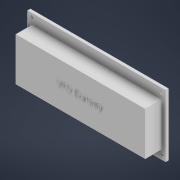
# Autodesk Inventor part: VFD_Dummy
Saved by Autodesk Inventor 2021.1 (Build 251245010, 245A)
## iProperties
Created: 2020-11-27
Part Number: VFD_Dummy
Material: Generic
Document SubType Name: Modeling
Designer: Alex
Density: 1 g/cm^3
Appearance: Default
Author: Alex
Autodesk Inventor part; units mm, degrees
ref_plane "YZ Plane" through (0, 0, 0) normal (1, 0, 0) x (0, 1, 0)
ref_plane "XZ Plane" through (0, 0, 0) normal (0, 1, 0) x (-1, 0, 0)
ref_plane "XY Plane" through (0, 0, 0) normal (0, 0, 1) x (1, 0, 0)
sketch "Sketch1" plane through (0, 0, 0) normal (0, 0, 1) x (1, 0, 0)
  line L0 (-40, 18) -> (40, 18)
  line L1 (40, 18) -> (40, -18)
  line L2 (40, -18) -> (-40, -18)
  line L3 (-40, -18) -> (-40, 18)
  point P0 (0, 0)
  point P1 (0, 18)
  point P2 (-40, 0)
  dimension "d0" = 36
  dimension "d1" = 80
  constraints: 8 end point, 2 midpoint, 2 parallel, 1 horizontal, 1 horizontal alignment, 1 perpendicular, 1 vertical alignment
  measures "d0" distance of L2.end L0.start
  measures "d1" distance of L0.start L0.end
extrude "Extrusion1" add sketch "Sketch1" along normal blind 1.6
sketch "Sketch2" plane through (0, 0, 1.6) normal (0, 0, 1) x (1, 0, 0)
  line L0 (-40, -18) -> (40, -18) construction
  line L1 (40, -18) -> (40, 18) construction
  line L2 (40, 18) -> (-40, 18) construction
  line L3 (-40, 18) -> (-40, -18) construction
  point P0 (0, 0)
  point P1 (-37.5, 15.5)
  point P2 (-37.5, -15.5)
  point P3 (37.5, -15.5)
  point P4 (37.5, 15.5)
  dimension "d4" = 2.5
  dimension "d5" = 2.5
  dimension "d6" = 2.5
  dimension "d7" = 2.5
  constraints: 2 horizontal alignment, 2 vertical alignment
  measures "d4" distance from line of L2 point (-37.5, 15.5)
  measures "d5" distance from line of L3 point (-37.5, 15.5)
  measures "d6" distance from line of L0 point (37.5, -15.5)
  measures "d7" distance from line of L1 point (37.5, -15.5)
hole "Hole1" at (-37.5, 15.5, 1.6) at (-37.5, -15.5, 1.6) at (37.5, -15.5, 1.6) at (37.5, 15.5, 1.6) direction (0, 0, -1) diameter 2.5 depth 5
sketch "Sketch3" plane through (0, 0, 1.6) normal (0, 0, 1) x (1, 0, 0)
  line L0 (-37.5, 11.95) -> (37.5, 11.95)
  line L1 (37.5, 11.95) -> (37.5, -13.05)
  line L2 (37.5, -13.05) -> (-37.5, -13.05)
  line L3 (-37.5, -13.05) -> (-37.5, 11.95)
  line L4 (-40, -18) -> (40, -18) projected
  point P0 (0, 0)
  point P1 (0, 11.95)
  dimension "d15" = 25
  dimension "d16" = 75
  dimension "d17" = 4.95
  constraints: 8 end point, 2 parallel, 1 horizontal, 1 midpoint, 1 perpendicular, 1 vertical alignment
  measures "d15" distance of L2.end L0.start
  measures "d16" distance of L0.start L0.end
  measures "d17" distance between parallel lines of L2 L4
extrude "Extrusion2" add sketch "Sketch3" along normal blind 9.35
sketch "Sketch4" plane through (0, 0, 10.95) normal (0, 0, 1) x (1, 0, 0)
  line L0 (-22.5, 4.45) -> (22.5, 4.45) construction
  line L1 (22.5, 4.45) -> (22.5, -5.55) construction
  line L2 (22.5, -5.55) -> (-22.5, -5.55) construction
  line L3 (-22.5, -5.55) -> (-22.5, 4.45) construction
  line L4 (-37.5, -13.05) -> (37.5, -13.05) construction
  line L5 (37.5, -13.05) -> (37.5, 11.95) construction
  line L6 (37.5, 11.95) -> (-37.5, 11.95) construction
  line L7 (-37.5, 11.95) -> (-37.5, -13.05) construction
  line L8 (37.5, 11.95) -> (-37.5, 11.95) construction
  line L9 (-10.3965, 1.6836) -> (-11.6019, -1.8164)
  line L10 (-11.6019, -1.8164) -> (-12.1039, -1.8164)
  line L11 (-12.1039, -1.8164) -> (-13.3094, 1.6836)
  line L12 (-13.3094, 1.6836) -> (-12.8102, 1.6836)
  line L13 (-12.8102, 1.6836) -> (-11.8402, -1.2236)
  line L14 (-11.8402, -1.2236) -> (-10.8701, 1.6836)
  line L15 (-10.8701, 1.6836) -> (-10.3965, 1.6836)
  line L16 (-7.9686, 1.2695) -> (-9.5966, 1.2695)
  line L17 (-9.5966, 1.2695) -> (-9.5966, 0.2825)
  line L18 (-9.5966, 0.2825) -> (-8.0367, 0.2825)
  line L19 (-8.0367, 0.2825) -> (-8.0367, -0.1316)
  line L20 (-8.0367, -0.1316) -> (-9.5966, -0.1316)
  line L21 (-9.5966, -0.1316) -> (-9.5966, -1.8164)
  line L22 (-9.5966, -1.8164) -> (-10.0618, -1.8164)
  line L23 (-10.0618, -1.8164) -> (-10.0618, 1.6836)
  line L24 (-10.0618, 1.6836) -> (-7.9686, 1.6836)
  line L25 (-7.9686, 1.6836) -> (-7.9686, 1.2695)
  spline S0 degree 2 poles (-4.7919, -0.0692) (-4.7919, -0.5486) (-5.1805, -1.3201) (-5.5067, -1.5356) knots 0 0 0 1 2 2 2
  spline S1 degree 2 poles (-5.5067, -1.5356) (-5.7733, -1.703) (-6.3207, -1.8164) (-6.7462, -1.8164) knots 0 0 0 1 2 2 2
  line L26 (-6.7462, -1.8164) -> (-7.5517, -1.8164)
  line L27 (-7.5517, -1.8164) -> (-7.5517, 1.6836)
  line L28 (-7.5517, 1.6836) -> (-6.7547, 1.6836)
  spline S2 degree 2 poles (-6.7547, 1.6836) (-6.2611, 1.6836) (-5.6996, 1.5361) (-5.501, 1.4056) knots 0 0 0 1 2 2 2
  spline S3 degree 2 poles (-5.501, 1.4056) (-5.1635, 1.1816) (-4.7919, 0.4413) (-4.7919, -0.0692) knots 0 0 0 1 2 2 2
  spline S4 degree 2 poles (-5.2769, -0.0636) (-5.2769, 0.3392) (-5.5436, 0.9093) (-5.8073, 1.0709) knots 0 0 0 1 2 2 2
  spline S5 degree 2 poles (-5.8073, 1.0709) (-5.9945, 1.1816) (-6.4171, 1.2808) (-6.732, 1.2808) knots 0 0 0 1 2 2 2
  line L29 (-6.732, 1.2808) -> (-7.0865, 1.2808)
  line L30 (-7.0865, 1.2808) -> (-7.0865, -1.4137)
  line L31 (-7.0865, -1.4137) -> (-6.732, -1.4137)
  spline S6 degree 2 poles (-6.732, -1.4137) (-6.4228, -1.4137) (-5.9548, -1.3144) (-5.7648, -1.1811) knots 0 0 0 1 2 2 2
  spline S7 degree 2 poles (-5.7648, -1.1811) (-5.5209, -1.0166) (-5.2769, -0.472) (-5.2769, -0.0636) knots 0 0 0 1 2 2 2
  spline S8 degree 2 poles (-0.0241, -0.0692) (-0.0241, -0.5486) (-0.4127, -1.3201) (-0.7389, -1.5356) knots 0 0 0 1 2 2 2
  spline S9 degree 2 poles (-0.7389, -1.5356) (-1.0055, -1.703) (-1.5529, -1.8164) (-1.9783, -1.8164) knots 0 0 0 1 2 2 2
  line L32 (-1.9783, -1.8164) -> (-2.7838, -1.8164)
  line L33 (-2.7838, -1.8164) -> (-2.7838, 1.6836)
  line L34 (-2.7838, 1.6836) -> (-1.9868, 1.6836)
  spline S10 degree 2 poles (-1.9868, 1.6836) (-1.4933, 1.6836) (-0.9317, 1.5361) (-0.7332, 1.4056) knots 0 0 0 1 2 2 2
  spline S11 degree 2 poles (-0.7332, 1.4056) (-0.3957, 1.1816) (-0.0241, 0.4413) (-0.0241, -0.0692) knots 0 0 0 1 2 2 2
  spline S12 degree 2 poles (-0.5091, -0.0636) (-0.5091, 0.3392) (-0.7757, 0.9093) (-1.0395, 1.0709) knots 0 0 0 1 2 2 2
  spline S13 degree 2 poles (-1.0395, 1.0709) (-1.2267, 1.1816) (-1.6493, 1.2808) (-1.9641, 1.2808) knots 0 0 0 1 2 2 2
  line L35 (-1.9641, 1.2808) -> (-2.3187, 1.2808)
  line L36 (-2.3187, 1.2808) -> (-2.3187, -1.4137)
  line L37 (-2.3187, -1.4137) -> (-1.9641, -1.4137)
  spline S14 degree 2 poles (-1.9641, -1.4137) (-1.655, -1.4137) (-1.187, -1.3144) (-0.997, -1.1811) knots 0 0 0 1 2 2 2
  spline S15 degree 2 poles (-0.997, -1.1811) (-0.753, -1.0166) (-0.5091, -0.472) (-0.5091, -0.0636) knots 0 0 0 1 2 2 2
  line L38 (2.4889, -1.8164) -> (2.0464, -1.8164)
  line L39 (2.0464, -1.8164) -> (2.0464, -1.5271)
  spline S16 degree 2 poles (2.0464, -1.5271) (1.8422, -1.7058) (1.4763, -1.8902) (1.2494, -1.8902) knots 0 0 0 1 2 2 2
  spline S17 degree 2 poles (1.2494, -1.8902) (1.0792, -1.8902) (0.7757, -1.7767) (0.6651, -1.6547) knots 0 0 0 1 2 2 2
  spline S18 degree 2 poles (0.6651, -1.6547) (0.5517, -1.5328) (0.4269, -1.1612) (0.4269, -0.8946) knots 0 0 0 1 2 2 2
  line L40 (0.4269, -0.8946) -> (0.4269, 0.81)
  line L41 (0.4269, 0.81) -> (0.8693, 0.81)
  line L42 (0.8693, 0.81) -> (0.8693, -0.6876)
  spline S19 degree 2 poles (0.8693, -0.6876) (0.8693, -0.8974) (0.9005, -1.1726) (0.9544, -1.2747) knots 0 0 0 1 2 2 2
  spline S20 degree 2 poles (0.9544, -1.2747) (1.0083, -1.3768) (1.1927, -1.4704) (1.3657, -1.4704) knots 0 0 0 1 2 2 2
  spline S21 degree 2 poles (1.3657, -1.4704) (1.5273, -1.4704) (1.8932, -1.286) (2.0464, -1.1527) knots 0 0 0 1 2 2 2
  line L43 (2.0464, -1.1527) -> (2.0464, 0.81)
  line L44 (2.0464, 0.81) -> (2.4889, 0.81)
  line L45 (2.4889, 0.81) -> (2.4889, -1.8164)
  line L46 (6.108, -1.8164) -> (6.108, -0.2962)
  spline S22 degree 2 poles (6.108, -0.2962) (6.108, -0.1146) (6.0796, 0.1945) (6.0342, 0.2796) knots 0 0 0 1 2 2 2
  spline S23 degree 2 poles (6.0342, 0.2796) (5.9889, 0.3732) (5.8158, 0.464) (5.6655, 0.464) knots 0 0 0 1 2 2 2
  spline S24 degree 2 poles (5.6655, 0.464) (5.5294, 0.464) (5.2174, 0.2966) (5.0529, 0.1378) knots 0 0 0 1 2 2 2
  spline S25 degree 2 poles (5.0529, 0.1378) (5.0557, 0.0981) (5.0614, -0.0125) (5.0614, -0.0863) knots 0 0 0 1 2 2 2
  line L47 (5.0614, -0.0863) -> (5.0614, -1.8164)
  line L48 (5.0614, -1.8164) -> (4.6189, -1.8164)
  line L49 (4.6189, -1.8164) -> (4.6189, -0.2962)
  spline S26 degree 2 poles (4.6189, -0.2962) (4.6189, -0.1146) (4.5906, 0.1945) (4.5452, 0.2796) knots 0 0 0 1 2 2 2
  spline S27 degree 2 poles (4.5452, 0.2796) (4.4998, 0.3732) (4.3268, 0.464) (4.1765, 0.464) knots 0 0 0 1 2 2 2
  spline S28 degree 2 poles (4.1765, 0.464) (4.0346, 0.464) (3.7198, 0.2853) (3.5723, 0.1463) knots 0 0 0 1 2 2 2
  line L50 (3.5723, 0.1463) -> (3.5723, -1.8164)
  line L51 (3.5723, -1.8164) -> (3.1299, -1.8164)
  line L52 (3.1299, -1.8164) -> (3.1299, 0.81)
  line L53 (3.1299, 0.81) -> (3.5723, 0.81)
  line L54 (3.5723, 0.81) -> (3.5723, 0.5207)
  spline S29 degree 2 poles (3.5723, 0.5207) (3.7453, 0.6937) (4.0857, 0.8838) (4.2899, 0.8838) knots 0 0 0 1 2 2 2
  spline S30 degree 2 poles (4.2899, 0.8838) (4.5225, 0.8838) (4.8827, 0.671) (4.9763, 0.4299) knots 0 0 0 1 2 2 2
  spline S31 degree 2 poles (4.9763, 0.4299) (5.1777, 0.654) (5.5577, 0.8838) (5.779, 0.8838) knots 0 0 0 1 2 2 2
  spline S32 degree 2 poles (5.779, 0.8838) (5.9491, 0.8838) (6.2271, 0.7788) (6.3292, 0.6597) knots 0 0 0 1 2 2 2
  spline S33 degree 2 poles (6.3292, 0.6597) (6.4342, 0.5406) (6.5504, 0.1832) (6.5504, -0.0863) knots 0 0 0 1 2 2 2
  line L55 (6.5504, -0.0863) -> (6.5504, -1.8164)
  line L56 (6.5504, -1.8164) -> (6.108, -1.8164)
  line L57 (10.1497, -1.8164) -> (10.1497, -0.2962)
  spline S34 degree 2 poles (10.1497, -0.2962) (10.1497, -0.1146) (10.1214, 0.1945) (10.076, 0.2796) knots 0 0 0 1 2 2 2
  spline S35 degree 2 poles (10.076, 0.2796) (10.0306, 0.3732) (9.8576, 0.464) (9.7073, 0.464) knots 0 0 0 1 2 2 2
  spline S36 degree 2 poles (9.7073, 0.464) (9.5711, 0.464) (9.2591, 0.2966) (9.0946, 0.1378) knots 0 0 0 1 2 2 2
  spline S37 degree 2 poles (9.0946, 0.1378) (9.0974, 0.0981) (9.1031, -0.0125) (9.1031, -0.0863) knots 0 0 0 1 2 2 2
  line L58 (9.1031, -0.0863) -> (9.1031, -1.8164)
  line L59 (9.1031, -1.8164) -> (8.6607, -1.8164)
  line L60 (8.6607, -1.8164) -> (8.6607, -0.2962)
  spline S38 degree 2 poles (8.6607, -0.2962) (8.6607, -0.1146) (8.6323, 0.1945) (8.5869, 0.2796) knots 0 0 0 1 2 2 2
  spline S39 degree 2 poles (8.5869, 0.2796) (8.5415, 0.3732) (8.3685, 0.464) (8.2182, 0.464) knots 0 0 0 1 2 2 2
  spline S40 degree 2 poles (8.2182, 0.464) (8.0764, 0.464) (7.7615, 0.2853) (7.6141, 0.1463) knots 0 0 0 1 2 2 2
  line L61 (7.6141, 0.1463) -> (7.6141, -1.8164)
  line L62 (7.6141, -1.8164) -> (7.1716, -1.8164)
  line L63 (7.1716, -1.8164) -> (7.1716, 0.81)
  line L64 (7.1716, 0.81) -> (7.6141, 0.81)
  line L65 (7.6141, 0.81) -> (7.6141, 0.5207)
  spline S41 degree 2 poles (7.6141, 0.5207) (7.7871, 0.6937) (8.1274, 0.8838) (8.3316, 0.8838) knots 0 0 0 1 2 2 2
  spline S42 degree 2 poles (8.3316, 0.8838) (8.5642, 0.8838) (8.9244, 0.671) (9.018, 0.4299) knots 0 0 0 1 2 2 2
  spline S43 degree 2 poles (9.018, 0.4299) (9.2194, 0.654) (9.5995, 0.8838) (9.8207, 0.8838) knots 0 0 0 1 2 2 2
  spline S44 degree 2 poles (9.8207, 0.8838) (9.9909, 0.8838) (10.2688, 0.7788) (10.3709, 0.6597) knots 0 0 0 1 2 2 2
  spline S45 degree 2 poles (10.3709, 0.6597) (10.4759, 0.5406) (10.5922, 0.1832) (10.5922, -0.0863) knots 0 0 0 1 2 2 2
  line L66 (10.5922, -0.0863) -> (10.5922, -1.8164)
  line L67 (10.5922, -1.8164) -> (10.1497, -1.8164)
  line L68 (13.2753, 0.81) -> (11.8628, -2.7836)
  line L69 (11.8628, -2.7836) -> (11.3892, -2.7836)
  line L70 (11.3892, -2.7836) -> (11.86, -1.6888)
  line L71 (11.86, -1.6888) -> (10.907, 0.81)
  line L72 (10.907, 0.81) -> (11.3835, 0.81)
  line L73 (11.3835, 0.81) -> (12.1011, -1.1357)
  line L74 (12.1011, -1.1357) -> (12.8158, 0.81)
  line L75 (12.8158, 0.81) -> (13.2753, 0.81)
  point P0 (0, 0)
  point P1 (-22.5, -0.55)
  point P2 (-37.5, -0.55)
  point P3 (0, 4.45)
  point P4 (0, 11.95)
  dimension "d20" = 45
  dimension "d21" = 10
  constraints: 4 midpoint, 1 horizontal, 1 horizontal alignment, 1 vertical alignment, 2 other
  measures "d20" distance of L0.start L0.end
  measures "d21" distance of L2.end L0.start
emboss "Emboss1" sketch "Sketch4" operation cut depth 1 direction (0, 0, -1)
equation "\"d5\" = d4"
equation "\"d6\" = d4"
equation "\"d7\" = d4"
body "Solid1"
